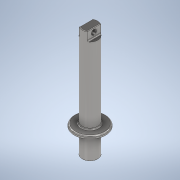
# Autodesk Inventor part: shield
Saved by Autodesk Inventor 2022 (Build 260153000, 153)
## iProperties
Created: 2021-07-20
Part Number: shield
Material: Steel, High Strength, Low Alloy
Document SubType Name: Modeling
Designer: Ian Kibandi
Density: 7.85 g/cm^3
Appearance: Steel - Polished
Author: Ian Kibandi
Autodesk Inventor part; units mm, degrees
ref_plane "YZ Plane" through (0, 0, 0) normal (1, 0, 0) x (0, 1, 0)
ref_plane "XZ Plane" through (0, 0, 0) normal (0, 1, 0) x (-1, 0, 0)
ref_plane "XY Plane" through (0, 0, 0) normal (0, 0, 1) x (1, 0, 0)
sketch "Sketch1" plane through (0, 0, 0) normal (0, 0, 1) x (1, 0, 0)
  line L0 (25, 0) -> (30, 0)
  line L1 (30, 0) -> (30, 100)
  line L2 (30, 100) -> (55, 100)
  line L3 (55, 100) -> (55, 95)
  line L4 (55, 95) -> (60, 95)
  line L5 (60, 95) -> (60, 105)
  line L6 (60, 105) -> (30, 105)
  line L7 (30, 105) -> (30, 395)
  line L8 (30, 395) -> (0, 395)
  line L9 (0, 250) -> (0, 395)
  line L10 (25, 0) -> (25, 250)
  line L11 (25, 250) -> (0, 250)
  line L12 (0, 0) -> (0, 395)
  dimension "d0" = 25
  dimension "d1" = 5
  dimension "d2" = 100
  dimension "d3" = 25
  dimension "d4" = 5
  dimension "d5" = 5
  dimension "d6" = 10
  dimension "d7" = 290
  dimension "d8" = 250
  constraints: 26 end point, 10 perpendicular, 2 point on line, 1 vertical
  measures "d0" distance of L12.start L0.start
  measures "d1" distance of L0.start L0.end
  measures "d2" distance of L0.end L1.end
  measures "d3" distance of L1.end L2.end
  measures "d4" distance of L2.end L3.end
  measures "d5" distance of L3.end L4.end
  measures "d6" distance of L4.end L5.end
  measures "d7" distance of L6.end L7.end
  measures "d8" distance of L0.start L10.end
revolve "Revolution1" add sketch "Sketch1" angle 360 mid plane about axis through (0, 0, 0) along (0, 1, 0)
fillet "Fillet1" radius 5 3 edges at (30, 105, 0) (60, 105, 0) (30, 100, 0)
sketch "Sketch2" plane through (0, 395, 0) normal (0, 1, 0) x (1, 0, 0)
  line L0 (15, 0) -> (-15, 0)
  circle A0 centre (0, 0) radius 25 projected
  circle A1 centre (0, 0) radius 30 projected
  line L1 (-15, -25.9808) -> (-15, 25.9808)
  line L2 (15, 0) -> (15, -25.9808)
  line L3 (15, -25.9808) -> (15, 25.9808)
  arc A2 (15, 25.9808) -> (-15, 25.9808) centre (0, 0) ccw
  arc A3 (-15, -25.9808) -> (15, -25.9808) centre (0, 0) ccw
  dimension "d11" = 15
  dimension "d12" = 30
  constraints: 8 end point, 8 point on circle, 2 centre point, 2 coincident, 1 horizontal, 1 vertical
  measures "d11" distance of point (0, 0) L0.start
  measures "d12" distance of L0.start L0.end
extrude "Extrusion1" add sketch "Sketch2" along normal blind 35 contours L2 A0 L1 L0 | L0 L1 A0 L3 | L2 A1 L1 A0 | A0 L1 A1 L3
fillet "Fillet2" radius 2 4 edges at (-15, 430, 0) (15, 430, 12.9904) (0, 430, -30) (0, 430, 30)
fillet "Fillet3" radius 5 2 edges at (-15, 395, 0) (15, 395, 12.9904)
sketch "Sketch3" plane through (-15, 428, -25.9808) normal (-1, 0, 0) x (0, 0, 1)
  line L0 (0, -28) -> (0, 0) projected
  line L1 (0, 0) -> (51.9615, 0) projected
  line L2 (0, -28) -> (51.9615, -28) projected
  circle A0 centre (25.9808, -14) radius 10
  point P0 (25.9808, -428)
  dimension "d17" = 20
  constraints: 1 centre point
  measures "d17" diameter of A0
hole "Hole1" at (-15, 414, 0) direction (1, 0, 0) diameter 20 end through all
fillet "Fillet4" radius 2 1 edges at (30, 0, 0)
body "Solid1"
